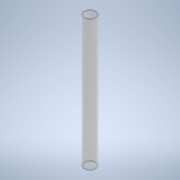
# Autodesk Inventor part: Barrel
Saved by Autodesk Inventor 2021 (Build 250183000, 183)
## iProperties
Created: 2020-03-16
Part Number: Barrel
Material: Generic
Document SubType Name: Modeling
Designer: Daniel
Density: 1 g/cm^3
Appearance: Light Gray Reflective
Author: Daniel
Autodesk Inventor part; units mm, degrees
ref_plane "YZ Plane" through (0, 0, 0) normal (1, 0, 0) x (0, 1, 0)
ref_plane "XZ Plane" through (0, 0, 0) normal (0, 1, 0) x (-1, 0, 0)
ref_plane "XY Plane" through (0, 0, 0) normal (0, 0, 1) x (1, 0, 0)
sketch "Sketch1" plane through (0, 0, 0) normal (0, 1, 0) x (-1, 0, 0)
  circle A0 centre (0, 0) radius 4.0831
  circle A1 centre (0, 0) radius 3.302
  dimension "d0" = 8.1661
  dimension "d1" = 6.604
  constraints: 2 centre point, 2 coincident
  measures "d0" diameter of A0
  measures "d1" diameter of A1
extrude "Extrusion1" add sketch "Sketch1" along normal blind 88.9
body "Solid1"
